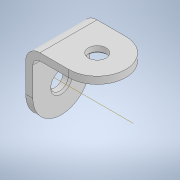
# Autodesk Inventor part: Angle Bracket
Saved by Autodesk Inventor 2022 (Build 260153000, 153)
## iProperties
Created: 2022-04-03
Part Number: Angle Bracket
Material: Generic
Document SubType Name: Modeling
Designer: Nick
Density: 1 g/cm^3
Appearance: Default
Author: Nick
Autodesk Inventor part; units mm, degrees
ref_plane "YZ Plane" through (0, 0, 0) normal (1, 0, 0) x (0, 1, 0)
ref_plane "XZ Plane" through (0, 0, 0) normal (0, 1, 0) x (-1, 0, 0)
ref_plane "XY Plane" through (0, 0, 0) normal (0, 0, 1) x (1, 0, 0)
sketch "Sketch1" plane through (0, 0, 0) normal (0, 0, 1) x (1, 0, 0)
  line L0 (0, 0) -> (0, 20.066)
  line L1 (0, 20.066) -> (20.066, 20.066)
  line L2 (20.066, 20.066) -> (20.066, 18.066)
  line L3 (20.066, 18.066) -> (2, 18.066)
  line L4 (2, 18.066) -> (2, 0)
  line L5 (2, 0) -> (0, 0)
  dimension "d0" = 20.066
  dimension "d1" = 20.066
  dimension "d2" = 2
  constraints: 12 end point, 2 horizontal, 2 perpendicular, 2 vertical, 1 parallel
  measures "d0" distance of L0.start L0.end
  measures "d1" distance of L0.end L1.end
  measures "d2" distance of L1.end L2.end
extrude "Extrusion1" add sketch "Sketch1" along normal blind 16.002
sketch "Sketch2" plane through (0, 0, 0) normal (-1, 0, 0) x (0, 0, 1)
  line L0 (16.002, 20.066) -> (16.002, 0) projected
  line L1 (0, 20.066) -> (16.002, 20.066) projected
  point P0 (0, 0)
  point P1 (8.001, 10.033)
  point P2 (16.002, 10.033)
  point P3 (8.001, 20.066)
  constraints: 2 midpoint, 1 horizontal alignment, 1 vertical alignment
sketch "Sketch5" plane through (2, 0, 0) normal (1, 0, 0) x (0, 0, -1)
  line L0 (0, 0) -> (0, 18.066) projected
  line L1 (0, 18.066) -> (-16.002, 18.066) projected
  line L2 (-16.002, 0) -> (-16.002, 18.066) projected
  line L3 (0, 0) -> (-16.002, 0) projected
  circle A0 centre (-8.001, 8.001) radius 8.001
  point P0 (0, 0)
  point P1 (0, 8.001)
  point P2 (-8.001, 0)
  point P3 (-16.002, 8.001)
  constraints: 3 tangent, 1 centre point
extrude "Extrusion3" cut sketch "Sketch5" against normal blind 16.002 contours L3 A0 L0 | L3 L2 A0
hole "Hole2" at (2, 8.001, 8.001) direction (-1, 0, 0) diameter 5 end through all countersink diameter 6 countersink angle 90 clearance for "Flat Head Machine Screw" size "M5" standard "Ansi Metric M Profile"
ref_plane "Work Plane1" through (2, 18.066, 0) normal (-0.7071068, -0.7071068, 0) x (0, 0, -1)
mirror "Mirror1" about plane through (2, 18.066, 0) normal (-0.7071068, -0.7071068, 0) of "Extrusion3", "Hole2"
fillet "Fillet1" radius 4 1 edges at (0, 20.066, 8.001)
fillet "Fillet2" radius 2 1 edges at (2, 18.066, 8.001)
equation "\"d1\" = d0"
body "Solid1"
